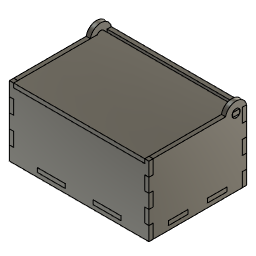
Box (Autodesk Fusion 360 design; units mm, degrees)
Autodesk Fusion 360 part; units mm, degrees
sketch "Sketch1" plane through (0, 0, 0) normal (0, 1, 0) x (1, 0, 0) in component "Front"
  line L0 (0, 0) -> (100, 0)
  line L1 (100, 0) -> (100, -50)
  line L2 (100, -50) -> (0, -50)
  line L3 (0, -50) -> (0, 0)
  line L4 (3, -50) -> (3, 0) construction
  line L5 (0, -3) -> (100, -3) construction
  line L6 (0, -6) -> (100, -6) construction
  line L7 (0, -10) -> (3, -10)
  line L8 (3, -10) -> (3, -20)
  line L9 (3, -20) -> (0, -20)
  line L10 (0, -20) -> (0, -10)
  line L11 (3, -20) -> (0, -20)
  line L12 (3, -30) -> (0, -30)
  line L13 (0, -30) -> (0, -40)
  line L14 (0, -40) -> (3, -40)
  line L15 (3, -40) -> (3, -30)
  line L16 (20, -3) -> (40, -3)
  line L17 (40, -3) -> (40, -6)
  line L18 (40, -6) -> (20, -6)
  line L19 (20, -6) -> (20, -3)
  line L20 (60, -6) -> (80, -6)
  line L21 (80, -6) -> (80, -3)
  line L22 (80, -3) -> (60, -3)
  line L23 (60, -3) -> (60, -6)
  line L24 (50, -50) -> (50, 0) construction
  line L25 (100, -40) -> (97, -40)
  line L26 (97, -50) -> (97, 0) construction
  line L27 (100, -10) -> (97, -10)
  line L28 (97, -30) -> (100, -30)
  line L29 (97, -20) -> (100, -20)
  line L30 (97, -10) -> (97, -20)
  line L31 (97, -20) -> (100, -20)
  line L32 (97, -40) -> (97, -30)
  dimension "d5" = 100
  dimension "d6" = 50
  dimension "d7" = 3
  dimension "d8" = 3
  dimension "d9" = 3
  dimension "d11" = 10
  dimension "d12" = 10
  dimension "d15" = 10
  dimension "d16" = 10
  dimension "d17" = 20
  dimension "d18" = 20
  dimension "d19" = 20
  dimension "d20" = 20
  dimension "d34" = 3
  constraint horizontal L0
  constraint vertical L1
  constraint horizontal L2
  constraint vertical L3
  constraint coincident L0.start L3.end
  constraint coincident L2 L4.start
  constraint coincident L0 L4.end
  constraint perpendicular L0 L4
  constraint coincident L3 L5.start
  constraint coincident L1 L5.end
  constraint perpendicular L1 L5
  constraint coincident L3 L6.start
  constraint coincident L1 L6.end
  constraint perpendicular L1 L6
  constraint horizontal L7
  constraint vertical L8
  constraint vertical L10
  constraint coincident L4 L8.end
  constraint coincident L3 L7.start
  constraint horizontal L11
  constraint horizontal L12
  constraint vertical L13
  constraint horizontal L14
  constraint vertical L15
  constraint coincident L3 L13.end
  constraint horizontal L16
  constraint vertical L17
  constraint horizontal L18
  constraint vertical L19
  constraint coincident L6 L17.end
  constraint coincident L5 L16.start
  constraint horizontal L20
  constraint vertical L21
  constraint horizontal L22
  constraint vertical L23
  constraint coincident L6 L20.start
  constraint midpoint L2 L24.start
  constraint midpoint L0 L24.end
  constraint symmetric L4.start L24 L26.start
  constraint symmetric L4.end L24 L26.end
  constraint symmetric L7.start L24 L27.start
  constraint symmetric L7.end L24 L27.end
  constraint symmetric L8.end L24 L29.start
  constraint symmetric L9.end L24 L29.end
  constraint symmetric L12.start L24 L28.start
  constraint symmetric L12.end L24 L28.end
  constraint symmetric L13.end L24 L25.start
  constraint symmetric L14.end L24 L25.end
  constraint collinear L26 L32
  measures "d5" distance of L1.end L2.end
  measures "d6" distance of L0.end L1.end
  measures "d7" distance of L3 L4
  measures "d8" distance of L0 L5
  measures "d9" distance of L5 L6
  measures "d11" distance of L0 L7
  measures "d12" distance of L7 L9
  measures "d15" distance of L11 L12
  measures "d16" distance of L12 L14
  measures "d17" distance of L3 L19
  measures "d18" distance of L17 L19
  measures "d19" distance of L17 L23
  measures "d20" distance of L21 L23
  measures "d34" distance of L0 L22
extrude "Extrude1" add sketch "Sketch1" along normal blind 3 contours L0 L1 L2 L3 L7 L8 L9 L11 L12 L14 L15 L25 L27 L28 L29 L30 L31 L32 makes body 1 in component "Front"
sketch "Sketch1 (2)" plane through (0, 0, 0) normal (-1, 0, 0) x (0, -1, 0) in component "Left"
  line L0 (0, 0) -> (0, 10)
  line L1 (0, 10) -> (-3, 10)
  line L2 (-3, 10) -> (-3, 0)
  line L3 (-3, 0) -> (0, 0)
  line L4 (0, 0) -> (-70, 0)
  line L5 (-70, 0) -> (-70, 50)
  line L6 (-70, 50) -> (0, 50)
  line L7 (0, 50) -> (0, 0)
  line L8 (0, 50) -> (-3, 50)
  line L9 (0, 3) -> (-70, 3)
  line L10 (0, 6) -> (-70, 6)
  line L11 (-14, 6) -> (-14, 3)
  line L12 (-28, 6) -> (-28, 3)
  line L13 (-42, 6) -> (-42, 3)
  line L14 (-56, 6) -> (-56, 3)
  circle A0 centre (-62.5, 48.5) radius 2.9155
  line L15 (-65, 50) -> (-60, 50)
  line L16 (-60, 50) -> (-60, 47)
  line L17 (-60, 47) -> (-65, 47)
  line L18 (-65, 47) -> (-65, 50)
  circle A1 centre (-62.5, 48.5) radius 7.6485
  dimension "d23" = 70
  dimension "d24" = 3
  dimension "d25" = 3
  dimension "d26" = 14
  dimension "d27" = 14
  dimension "d28" = 14
  dimension "d29" = 14
  dimension "d39" = 3
  dimension "d40" = 5
  dimension "d44" = 5
  constraint horizontal L4
  constraint vertical L5
  constraint horizontal L6
  constraint vertical L7
  constraint coincident L0.start L3.end
  constraint collinear L6 L8
  constraint coincident L7 L9.start
  constraint coincident L5 L9.end
  constraint perpendicular L5 L9
  constraint coincident L7 L10.start
  constraint coincident L5 L10.end
  constraint perpendicular L5 L10
  constraint coincident L10 L11.start
  constraint coincident L9 L11.end
  constraint perpendicular L9 L11
  constraint coincident L10 L12.start
  constraint coincident L9 L12.end
  constraint perpendicular L9 L12
  constraint coincident L10 L13.start
  constraint coincident L9 L13.end
  constraint perpendicular L9 L13
  constraint coincident L10 L14.start
  constraint coincident L9 L14.end
  constraint perpendicular L9 L14
  constraint horizontal L15
  constraint vertical L16
  constraint horizontal L17
  constraint vertical L18
  constraint coincident A0 L16.end
  constraint coincident A0 L15.start
  constraint coincident A0 L17.end
  constraint collinear L6 L15
  constraint concentric A0 A1
  constraint coincident L5.end A1
  measures "d23" distance of L5.end L6.end
  measures "d24" distance of L4 L9
  measures "d25" distance of L9 L10
  measures "d26" distance of L7 L11
  measures "d27" distance of L11 L12
  measures "d28" distance of L12 L13
  measures "d29" distance of L13 L14
  measures "d39" distance of L15.start L17.end
  measures "d40" distance of L15.start L15.end
  measures "d44" distance of L5.end L15.start
extrude "Extrude1'" add sketch "Sketch1 (2)" against normal blind 3 separate body contours L0 L2 L3 L4 L7 L9 | L0 L2 L7 L9 L10 | L2 L4 L5 L9 | L0 L1 L2 L7 L10 | L2 L9 L10 L11 | L1 L2 L5 L6 L7 L8 L10 A1 | L5 L9 L10 L14 | L9 L10 L12 L13 | L5 L6 A0 A1 | L6 A0 A1 makes body 2 in component "Left"
combine "Combine1" operation cut target body 2 tool bodies 1 keep tools in component "Left"
ref_plane "WorkPlane1" through (50, 1.5, 5) normal (-1, 0, 0) x (0, 0, 1)
mirror "MirrorComponent1" about plane through (0, 0, 0) normal (0, 0, 1) of bodies 2 makes body 3 in component "Left(Mirror)"
ref_plane "WorkPlane2" through (1.5, 35, 25) normal (0, -1, 0) x (0, 0, -1)
mirror "MirrorComponent2" about plane through (0, 0, 0) normal (0, 0, 1) of bodies 1 makes body 4 in component "Front(Mirror)"
combine "Combine2" operation cut target body 2 tool bodies 4 body 4 seen with x (1, 0, 0) y (0, -1, 0) z (0, 0, -1) at (0, 70, 0) keep tools in component "Left"
combine "Combine1'" operation cut target body 3 tool bodies 4 body 4 seen with x (-1, 0, 0) y (0, -1, 0) z (0, 0, 1) at (100, 70, 0) keep tools in component "Left(Mirror)"
sketch "Sketch1 (3)" plane through (0, 0, 3) normal (0, 0, 1) x (-1, 0, 0) in component "Base"
  line L0 (-20, 0) -> (-40, 0)
  line L1 (-40, 0) -> (-40, -3)
  line L2 (-40, -3) -> (-20, -3)
  line L3 (-20, -3) -> (-20, 0)
  line L4 (0, 0) -> (-100, 0)
  line L5 (-100, 0) -> (-100, -70)
  line L6 (-100, -70) -> (0, -70)
  line L7 (0, -70) -> (0, 0)
  line L8 (-100, -70) -> (0, -70)
  line L9 (-100, -3) -> (-100, -55)
  constraint horizontal L4
  constraint vertical L5
  constraint horizontal L6
  constraint vertical L7
  constraint coincident L4.start L7.end
  constraint collinear L6 L8
  constraint collinear L5 L9
extrude "Extrude1''" add sketch "Sketch1 (3)" along normal blind 3 separate body makes body 5 in component "Base"
combine "Combine1''" operation cut target body 5 tool bodies 2 3 1 4 body 3 seen with x (-1, 0, 0) y (0, 1, 0) z (0, 0, -1) at (100, 0, 0) body 4 seen with x (1, 0, 0) y (0, -1, 0) z (0, 0, -1) at (0, 70, 0) keep tools in component "Base"
sketch "Sketch2" plane through (0, 0, 50) normal (0, 0, 1) x (-1, 0, 0) in component "Front"
  line L0 (0, 0) -> (-100, 0)
  line L1 (-100, 0) -> (-100, -3)
  line L2 (-100, -3) -> (0, -3)
  line L3 (0, -3) -> (0, 0)
  line L4 (-3, -3) -> (-97, -3)
  line L5 (-97, -3) -> (-97, 0)
  line L6 (-97, 0) -> (-3, 0)
  line L7 (-3, 0) -> (-3, -3)
  dimension "d35" = 3
  dimension "d36" = 3
  constraint horizontal L4
  constraint vertical L5
  constraint horizontal L6
  constraint vertical L7
  constraint coincident L0 L5.end
  constraint coincident L2 L4.start
  measures "d35" distance of L1 L4.end
  measures "d36" distance of L3 L7
extrude "Extrude2" cut sketch "Sketch2" against normal blind 3 contours L0 L2 L4 L5 L6 L7 bodies 1 in component "Front"
sketch "Sketch1 (4)" plane through (0, 0, 50) normal (0, 0, 1) x (-1, 0, 0) in component "Lid"
  line L0 (0, -3) -> (-3, -3)
  line L1 (-3, -3) -> (-3, -55)
  line L2 (-3, -55) -> (0, -55)
  line L3 (0, -55) -> (0, -3)
  line L4 (-3, 0) -> (-97, 0)
  line L5 (-97, 0) -> (-97, -65)
  line L6 (-97, -65) -> (-3, -65)
  line L7 (-3, -65) -> (-3, 0)
  line L8 (-3, 0) -> (0, 0)
  line L9 (-100, -70) -> (0, -70)
  line L10 (-97, -65) -> (-100, -65)
  line L11 (-100, -65) -> (-100, -60)
  line L12 (-100, -60) -> (-97, -60)
  line L13 (-97, -60) -> (-97, -65)
  line L14 (-100, -3) -> (-100, -67)
  line L15 (-3, -65) -> (0, -65)
  line L16 (0, -65) -> (0, -60)
  line L17 (0, -60) -> (-3, -60)
  line L18 (-3, -60) -> (-3, -65)
  line L19 (0, -3) -> (0, -67)
  point P0 (-97, 0)
  dimension "d43" = 5
  dimension "d45" = 5
  dimension "d46" = 5
  constraint horizontal L4
  constraint vertical L5
  constraint horizontal L6
  constraint vertical L7
  constraint coincident L4.start L8
  constraint coincident L7 L4.start
  constraint coincident P0 L4.end
  constraint horizontal L10
  constraint vertical L11
  constraint horizontal L12
  constraint vertical L13
  constraint collinear L11 L14
  constraint horizontal L15
  constraint vertical L16
  constraint horizontal L17
  constraint vertical L18
  constraint collinear L16 L19
  measures "d43" distance of L6 L9
  measures "d45" distance of L10 L12
  measures "d46" distance of L15 L17
extrude "Extrude1'''" add sketch "Sketch1 (4)" against normal blind 3 separate body contours L1 L4 L5 L6 L7 L13 L18 | L7 L15 L16 L17 L18 L19 | L5 L10 L11 L12 L13 L14 makes body 6 in component "Lid"
component "Front" placed x (1, 0, 0) y (0, 1, 0) z (0, 0, 1) at (0, 0, 0)
component "Left" placed x (1, 0, 0) y (0, 1, 0) z (0, 0, 1) at (0, 0, 0)
component "Base" placed x (1, 0, 0) y (0, 1, 0) z (0, 0, 1) at (0, 0, 0)
component "Lid" placed x (1, 0, 0) y (0, 1, 0) z (0, 0, 1) at (0, 0, 0)
component "Left(Mirror)" placed x (-1, 0, 0) y (0, 1, 0) z (0, 0, -1) at (100, 0, 0)
component "Front(Mirror)" placed x (1, 0, 0) y (0, -1, 0) z (0, 0, -1) at (0, 70, 0)
equation "L = 100 mm" comment "Length"
equation "w = 70 mm" comment "Width"
equation "h = 50 mm" comment "Height"
equation "t = 3 mm" comment "Wood Thickness"
equation "d5 = L"
equation "d6 = h"
equation "d7 = t"
equation "d8 = t"
equation "d9 = t"
equation "nt = 2" comment "Number of Tabs"
equation "d11 = h / ( 2 * nt + 1 )"
equation "d12 = d11"
equation "d15 = d12"
equation "d16 = d15"
equation "d17 = L / ( 2 * nt + 1 )"
equation "d18 = d17"
equation "d19 = d18"
equation "d20 = d19"
equation "d21 = t"
equation "d23 = w"
equation "d24 = t"
equation "d25 = t"
equation "d26 = d23 / ( 2 * nt + 1 )"
equation "d27 = d26"
equation "d28 = d27"
equation "d29 = d28"
equation "d30 = -t"
equation "d32 = t"
equation "d34 = t"
equation "d35 = t"
equation "d36 = t"
equation "d37 = -t"
equation "d39 = t"
equation "d47 = -t"
